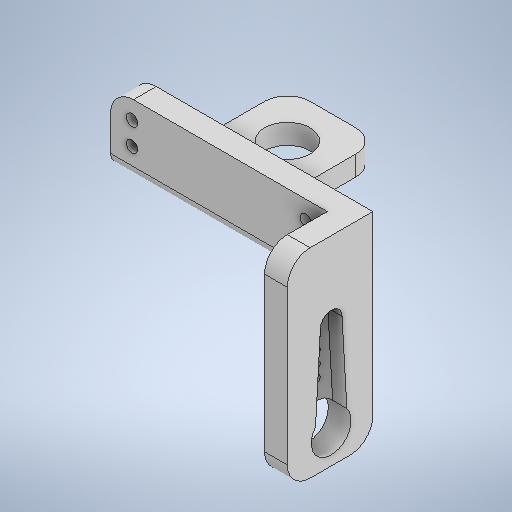
# Autodesk Inventor part: end-effector
Saved by Autodesk Inventor 2025 (Build 290162000, 162)
## iProperties
Created: 2024-07-13
Part Number: end-effector
Material: Generic
Document SubType Name: Modeling
Designer: hifzhil
Density: 1 g/cm^3
Appearance: Default
Author: hifzhil
## iProperties of the stored document end-effector_3DPrint.ipt
Created: 2024-07-13
Part Number: end-effector_3DPrint
Material: Generic
Document SubType Name: Modeling
Designer: hifzhil
Density: 1 g/cm^3
Appearance: Default
Author: hifzhil
Autodesk Inventor part; units mm, degrees
ref_plane "YZ Plane" through (0, 0, 0) normal (1, 0, 0) x (0, 1, 0)
ref_plane "XZ Plane" through (0, 0, 0) normal (0, 1, 0) x (-1, 0, 0)
ref_plane "XY Plane" through (0, 0, 0) normal (0, 0, 1) x (1, 0, 0)
sketch "Sketch1" plane through (0, 0, 0) normal (0, 0, 1) x (1, 0, 0)
  line L0 (-19, 7.0885) -> (19, 7.0885)
  line L1 (19, 7.0885) -> (19, -7.0885)
  line L2 (19, -7.0885) -> (-19, -7.0885)
  line L3 (-19, -7.0885) -> (-19, 7.0885)
  point P0 (0, 0)
  point P1 (0, -7.0885)
  point P2 (-19, 0)
  dimension "d13" = 38
  constraints: 8 end point, 2 midpoint, 1 horizontal alignment, 1 parallel, 1 perpendicular, 1 vertical alignment
  measures "d13" distance of L0.start L0.end
extrude "Extrusion1" add sketch "Sketch1" along normal blind 4
ref_plane "Work Plane1" through (0, 0, 4) normal (0, 0, 1) x (1, 0, 0)
sketch "Sketch2" plane through (0, 0, 4) normal (0, 0, 1) x (1, 0, 0)
  circle A0 centre (-15.25, 3.8656) radius 1
  circle A1 centre (-15.25, -0.1344) radius 1
  circle A2 centre (15.25, 3.8656) radius 1
  circle A3 centre (15.25, -0.1344) radius 1
  point P0 (0, 0)
  dimension "d3" = 2
  dimension "d4" = 2
  dimension "d5" = 2
  dimension "d6" = 2
  dimension "d7" = 30.5
  dimension "d8" = 30.5
  dimension "d9" = 4
  dimension "d10" = 4
  dimension "d11" = 15.25
  dimension "d12" = 15.25
  constraints: 4 centre point
  measures "d3" diameter of A0
  measures "d4" diameter of A1
  measures "d5" diameter of A2
  measures "d6" diameter of A3
  measures "d7" distance of A3.centre A1.centre
  measures "d8" distance of A2.centre A0.centre
  measures "d9" distance of A1.centre A0.centre
  measures "d10" distance of A3.centre A2.centre
  measures "d11" horizontal distance of A1.centre point (0, 0)
  measures "d12" horizontal distance of point (0, 0) A0.centre
ref_plane "Work Plane2" through (0, 0, 0) normal (0, 0, -1) x (-1, 0, 0)
sketch "Sketch3" plane through (0, 0, 0) normal (0, 0, -1) x (-1, 0, 0)
  line L0 (-8, 2.3239) -> (8, 2.3239)
  line L1 (8, 2.3239) -> (8, -1.1761)
  line L2 (8, -1.1761) -> (-8, -1.1761)
  line L3 (-8, -1.1761) -> (-8, 2.3239)
  point P0 (0, 0)
  point P1 (0, -1.1761)
  dimension "d15" = 3.5
  dimension "d16" = 16
  constraints: 8 end point, 2 parallel, 1 horizontal, 1 midpoint, 1 perpendicular, 1 vertical alignment
  measures "d15" distance of L2.end L0.start
  measures "d16" distance of L0.start L0.end
extrude "Extrusion2" add sketch "Sketch3" along normal blind 16
ref_plane "Work Plane3" through (-8, 2.3239, 0) normal (0, 1, 0) x (1, 0, 0)
sketch "Sketch4" plane through (-8, 2.3239, 0) normal (0, 1, 0) x (1, 0, 0)
  circle A0 centre (8, 8) radius 4
  line L0 (0, 0) -> (0, 16) projected
  line L1 (0, 16) -> (16, 16) projected
  point P0 (8, 0)
  point P1 (0, 8)
  dimension "d20" = 8
  dimension "d21" = 8
  dimension "d22" = 8
  constraints: 1 centre point, 1 midpoint
  measures "d20" diameter of A0
  measures "d21" distance of point (0, 8) A0.centre
  measures "d22" distance from line of L1 A0.centre
extrude "Extrusion3" cut sketch "Sketch4" against normal blind 4
fillet "Fillet1" radius 4 2 edges at (-8, 0.5739, -16) (8, 0.5739, -16)
ref_plane "Work Plane4" through (19, -7.0885, 0) normal (1, 0, 0) x (0, 0, -1)
sketch "Sketch5" plane through (19, -7.0885, 0) normal (1, 0, 0) x (0, 0, -1)
  point P0 (0, 7.0885)
sketch "Sketch6" plane through (19, -7.0885, 0) normal (1, 0, 0) x (0, 0, -1)
  line L0 (0, 14.1769) -> (0, 0) projected
  line L1 (0, 14.1769) -> (-15, 14.1769)
  line L2 (-15, 14.1769) -> (-15, -20.8231)
  line L3 (-15, -20.8231) -> (0, -20.8231)
  line L4 (0, -20.8231) -> (0, 14.1769)
  point P0 (0, 7.0885)
  dimension "d29" = 15
  dimension "d30" = 35
  constraints: 8 end point, 2 parallel, 1 horizontal, 1 perpendicular
  measures "d29" distance of L2.end L3.end
  measures "d30" distance of L1.end L2.end
extrude "Extrusion4" add sketch "Sketch6" along normal blind 4
ref_plane "Work Plane5" through (19, -7.0885, 0) normal (-1, 0, 0) x (0, 0, 1)
ref_plane "Work Plane7" through (23, -7.0885, 0) normal (1, 0, 0) x (0, 0, -1)
ref_plane "Work Plane8" through (23, -7.0885, 0) normal (1, 0, 0) x (0, 0, -1)
ref_plane "Work Plane9" through (23, -7.0885, 0) normal (1, 0, 0) x (0, 0, -1)
ref_plane "Work Plane10" through (-19, -7.0885, 0) normal (0, -1, 0) x (1, 0, 0)
extrude "Extrusion9" cut sketch "Sketch2" against normal blind 4
sketch "Sketch12" plane through (-19, -7.0885, 0) normal (0, -1, 0) x (1, 0, 0)
  line L0 (38, 4) -> (0, 4) projected
  line L1 (38, 4) -> (3, 4)
  line L2 (3, 4) -> (3, 0)
  line L3 (3, 0) -> (38, 0)
  line L4 (38, 0) -> (38, 4)
  point P0 (19, 0)
  point P1 (3, 4)
  constraints: 8 end point, 2 parallel, 1 horizontal, 1 perpendicular
extrude "Extrusion10" cut sketch "Sketch12" against normal blind 2
ref_plane "Work Plane11" through (23, -7.0885, 0) normal (1, 0, 0) x (0, 0, -1)
sketch "Sketch13" plane through (23, -7.0885, 0) normal (1, 0, 0) x (0, 0, -1)
  circle A0 centre (-7.3075, -15.6371) radius 3.5
  line L0 (-9.2075, 0.9629) -> (-10.0575, -13.472)
  arc A1 (-5.4075, 0.9629) -> (-9.2075, 0.9629) centre (-7.3075, 0.9629) ccw
  line L1 (-4.9308, -7.132) -> (-4.5575, -13.472)
  line L2 (-4.5575, -13.472) -> (-5.4075, 0.9629)
  circle A2 centre (-7.3075, -8.8371) radius 0.6
  circle A3 centre (-7.3075, -8.8371) radius 0.6
  circle A4 centre (-7.3075, -6.7371) radius 0.6
  circle A5 centre (-7.3075, -6.7371) radius 0.6
  circle A6 centre (-7.3075, -4.6371) radius 0.6
  circle A7 centre (-7.3075, -4.6371) radius 0.6
  circle A8 centre (-7.3075, -2.5371) radius 0.6
  circle A9 centre (-7.3075, -2.5371) radius 0.6
  circle A10 centre (-7.3075, -0.4371) radius 0.6
  circle A11 centre (-7.3075, -0.4371) radius 0.6
  circle A12 centre (-7.3075, 1.6629) radius 0.6
  circle A13 centre (-7.3075, 1.6629) radius 0.6
  point P0 (0, 7.0885)
  constraints: 14 centre point, 7 coincident, 6 end point, 2 point on circle, 1 collinear
ref_plane "Work Plane12" through (23, -7.0885, 0) normal (1, 0, 0) x (0, 0, -1)
sketch "Sketch14" plane through (23, -7.0885, 0) normal (1, 0, 0) x (0, 0, -1)
  circle A0 centre (-7.3075, -15.6371) radius 3.5
  line L0 (-9.2075, 0.9629) -> (-10.0575, -13.472)
  arc A1 (-5.4075, 0.9629) -> (-9.2075, 0.9629) centre (-7.3075, 0.9629) ccw
  line L1 (-4.9308, -7.1319) -> (-4.5575, -13.472)
  line L2 (-4.5575, -13.472) -> (-5.4075, 0.9629)
  circle A2 centre (-7.3075, -8.8371) radius 0.6
  circle A3 centre (-7.3075, -8.8371) radius 0.6
  circle A4 centre (-7.3075, -6.7371) radius 0.6
  circle A5 centre (-7.3075, -6.7371) radius 0.6
  circle A6 centre (-7.3075, -4.6371) radius 0.6
  circle A7 centre (-7.3075, -4.6371) radius 0.6
  circle A8 centre (-7.3075, -2.5371) radius 0.6
  circle A9 centre (-7.3075, -2.5371) radius 0.6
  circle A10 centre (-7.3075, -0.4371) radius 0.6
  circle A11 centre (-7.3075, -0.4371) radius 0.6
  circle A12 centre (-7.3075, 1.6629) radius 0.6
  circle A13 centre (-7.3075, 1.6629) radius 0.6
  point P0 (0, 7.0885)
  point P1 (0, 6.5288)
  constraints: 14 centre point, 7 coincident, 6 end point, 2 point on circle, 1 collinear
ref_plane "Work Plane13" through (23, -7.0885, 0) normal (1, 0, 0) x (0, 0, -1)
sketch "Sketch15" plane through (23, -7.0885, 0) normal (1, 0, 0) x (0, 0, -1)
  line L0 (-9.2075, 0.9629) -> (-10.0575, -13.472)
  arc A0 (-5.4075, 0.9629) -> (-9.2075, 0.9629) centre (-7.3075, 0.9629) ccw
  line L1 (-4.9308, -7.132) -> (-4.5575, -13.472)
  line L2 (-4.5575, -13.472) -> (-5.4075, 0.9629)
  circle A1 centre (-7.3075, -8.8371) radius 0.6
  circle A2 centre (-7.3075, -8.8371) radius 0.6
  circle A3 centre (-7.3075, -6.7371) radius 0.6
  circle A4 centre (-7.3075, -6.7371) radius 0.6
  circle A5 centre (-7.3075, -4.6371) radius 0.6
  circle A6 centre (-7.3075, -4.6371) radius 0.6
  circle A7 centre (-7.3075, -2.5371) radius 0.6
  circle A8 centre (-7.3075, -2.5371) radius 0.6
  circle A9 centre (-7.3075, -0.4371) radius 0.6
  circle A10 centre (-7.3075, -0.4371) radius 0.6
  circle A11 centre (-7.3075, 1.6629) radius 0.6
  circle A12 centre (-7.3075, 1.6629) radius 0.6
  arc A13 (-4.5575, -13.472) -> (-10.0575, -13.472) centre (-7.3075, -15.6371) ccw
  point P0 (0, 7.0885)
  point P1 (0, 6.5288)
  point P2 (0, 6.5288)
  point P3 (-7.3075, -15.6371)
  dimension "d52" = 3.5
  constraints: 14 centre point, 6 coincident, 6 end point, 4 point on circle, 1 collinear
  measures "d52" radius of A13
extrude "Extrusion11" cut sketch "Sketch13" against normal blind 2.5 contours A0 L0 A1 L2 L1 | A2 | A4 | A6 | A8 | A10 | A12
extrude "Extrusion12" cut sketch "Sketch14" against normal blind 4 contours A0
extrude "Extrusion13" cut sketch "Sketch15" against normal blind 4 contours A1 | A3 | A5 | A7 | A9 | A11
ref_plane "Work Plane14" through (-19, -7.0885, 0) normal (0, -1, 0) x (1, 0, 0)
sketch "Sketch16" plane through (-19, -7.0885, 0) normal (0, -1, 0) x (1, 0, 0)
  line L0 (38, 4) -> (0, 4) projected
  line L1 (0, 4) -> (3.3578, 4)
  line L2 (3.3578, 4) -> (3.3578, 0)
  line L3 (3.3578, 0) -> (0, 0)
  line L4 (0, 0) -> (0, 4)
  point P0 (19, 0)
  point P1 (3.3578, 4)
  constraints: 8 end point, 2 parallel, 1 horizontal, 1 perpendicular
extrude "Extrusion14" cut sketch "Sketch16" against normal blind 2
fillet "Fillet2" radius 2 2 edges at (0, -5.0885, 4) (0, -5.0885, 0)
fillet "Fillet3" radius 4 2 edges at (21, -27.9115, 15) (21, -27.9115, 0)
fillet "Fillet4" radius 4 1 edges at (21, 7.0885, 15)
fillet "Fillet5" radius 4 1 edges at (-19, 7.0885, 2)
body "Solid1"
